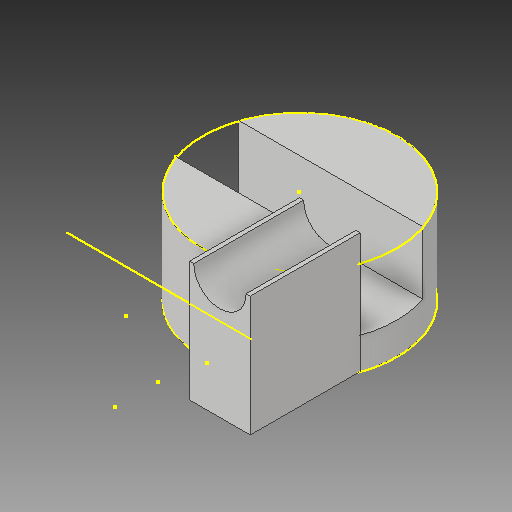
# Autodesk Inventor part: cilindro
Saved by Autodesk Inventor 2018.2 (Build 222227000, 227)
## iProperties
Created: 2016-04-06
Part Number: cilindro
Material: Genérico
Document SubType Name: Modeling
Designer: Usuario
Density: 1 g/cm^3
Appearance: Valor por defecto
Author: Usuario
Autodesk Inventor part; units mm, degrees
ref_plane "YZ Plane" through (0, 0, 0) normal (1, 0, 0) x (0, 1, 0)
ref_plane "XZ Plane" through (0, 0, 0) normal (0, 1, 0) x (-1, 0, 0)
ref_plane "XY Plane" through (0, 0, 0) normal (0, 0, 1) x (1, 0, 0)
sketch "Boceto1" plane through (0, 0, 0) normal (0, 1, 0) x (-1, 0, 0)
  circle A0 centre (0, 0) radius 46.5
  dimension "d0" = 93
  constraints: 1 centre point, 1 coincident
  measures "d0" diameter of A0
extrude "Extrusión1" add sketch "Boceto1" along normal blind 45
sketch "Boceto2" plane through (0, 0, 0) normal (0, -1, 0) x (1, 0, 0)
  point P0 (0, 0)
sketch "Boceto3" plane through (0, 45, 0) normal (0, 1, 0) x (1, 0, 0)
  line L0 (46.5, -15) -> (-46.6883, -15)
  circle A0 centre (0, 0) radius 46.5 projected
  line L1 (46.5, -15) -> (46.5, 15)
  line L2 (46.5, 0) -> (46.5, -15)
  line L3 (46.5, 0) -> (46.5, 15)
  line L4 (-46.6883, -15) -> (-46.6883, 15)
  line L5 (-46.6883, 15) -> (46.5, 15)
  constraints: 13 end point, 2 midpoint, 2 vertical, 1 horizontal, 1 horizontal alignment, 1 perpendicular, 1 point on line, 1 other
extrude "Extrusión2" cut sketch "Boceto3" against normal blind 30 contours L0 A0 L1 | L0 A0 L5 | A0 L5 L1 | L0 L4 L5 A0
sketch "Boceto4" plane through (0, 45, 0) normal (0, 1, 0) x (1, 0, 0)
  circle A0 centre (0, 0) radius 46.5 projected
  point P0 (-44.0142, -15)
  point P1 (44.0142, -15)
sketch "Boceto5" plane through (0, 45, 0) normal (0, 1, 0) x (1, 0, 0)
  line L0 (-20.0239, -77.8543) -> (-20, -77.821)
  point P0 (0, 0)
  point P1 (-20, -41.9792)
  point P2 (0, 0)
  point P3 (0, 0)
  constraints: 2 end point
extrude "Extrusión3" [suppressed]
sketch "Boceto6" plane through (0, 45, 0) normal (0, 1, 0) x (1, 0, 0)
  point P0 (0, 0)
sketch "Boceto7" plane through (0, 45, 0) normal (0, 1, 0) x (1, 0, 0)
  point P0 (0, 0)
sketch "Boceto8" plane through (0, 45, 0) normal (0, 1, 0) x (1, 0, 0)
  point P0 (0, 0)
sketch "Boceto9" plane through (0, 0, 0) normal (0, -1, 0) x (1, 0, 0)
  arc A0 (-44.0142, -15) -> (-44.0142, 15) centre (0, 0) ccw projected
  point P0 (5, 46.2304)
  point P1 (19.0142, 42.4348)
hole "Agujero1" at (0, 0, 0) direction (0, 1, 0) diameter 3.5 depth 10
sketch "Boceto10" plane through (0, 0, 0) normal (0, -1, 0) x (1, 0, 0)
  point P0 (0, 0)
sketch "Boceto11" plane through (0, 0, 0) normal (0, -1, 0) x (1, 0, 0)
  point P0 (0, 0)
sketch "Boceto12" plane through (0, 0, 0) normal (0, -1, 0) x (1, 0, 0)
  line L0 (1.5, -0.9014) -> (-1.5, -0.9014)
  arc A0 (-1.5, -0.9014) -> (1.5, -0.9014) centre (0, 0) ccw
  constraints: 2 end point, 2 point on circle, 1 centre point, 1 coincident
extrude "Extrusión4" add sketch "Boceto12" against normal blind 10
sketch "Boceto13" plane through (5, 40, 88) normal (0, 0, 1) x (1, 0, 0)
  point P0 (-5, -40)
  point P1 (39.0142, 0)
sketch "Boceto14" plane through (5, 40, 88) normal (0, 0, 1) x (1, 0, 0)
  point P0 (-5, -40)
sketch "Boceto15" plane through (5, 40, 88) normal (0, 0, 1) x (1, 0, 0)
  point P0 (-5, -40)
  point P1 (39.0142, 0)
sketch "Boceto16" plane through (5, 40, 88) normal (0, 0, 1) x (1, 0, 0)
  point P0 (-5, -40)
  point P1 (0, 0)
  point P2 (39.0142, 0)
sketch "Boceto17" plane through (5, 40, 88) normal (0, 0, 1) x (1, 0, 0)
  point P0 (-5, -40)
  point P1 (39.0586, 0)
  point P2 (0, 0)
sketch "Boceto18" plane through (5, 40, 88) normal (0, 0, 1) x (1, 0, 0)
  line L0 (0, -40) -> (0, 0) projected
  line L1 (39.0142, -40) -> (0, -40) projected
  line L2 (39.0142, 20) -> (39.0142, -40)
  line L3 (0, 20) -> (0, -40)
  line L4 (0, -40) -> (39.0142, -40)
  line L5 (0, 20) -> (2, 20)
  line L6 (39.0142, 20) -> (38, 20)
  arc A0 (2, 20) -> (38, 20) centre (20, 18.1) ccw
  point P0 (-5, -40)
  constraints: 10 end point, 2 horizontal, 2 perpendicular, 2 point on circle, 1 centre point
extrude "Extrusión5" [suppressed]
sketch "Boceto19" plane through (0, 15, 0) normal (0, 1, 0) x (1, 0, 0)
  point P0 (0, 0)
sketch "Boceto20" plane through (0, 45, 0) normal (0, 1, 0) x (1, 0, 0)
  point P0 (0, 0)
sketch "Boceto21" plane through (0, 45, 0) normal (0, 1, 0) x (1, 0, 0)
  point P0 (0, 0)
sketch "Boceto22" plane through (0, 45, 0) normal (0, 1, 0) x (1, 0, 0)
  point P0 (0, 0)
sketch "Boceto23" plane through (19.0142, 40, 67.4096) normal (0, 0, 1) x (1, 0, 0)
  line L0 (25, 0) -> (-63.0284, 0) projected
  point P0 (-19.0142, -40)
sketch "Boceto24" plane through (0, 45, 0) normal (0, 1, 0) x (1, 0, 0)
  arc A0 (-1.5, 0.9014) -> (1.5, 0.9014) centre (0, 0) ccw projected
  arc A1 (15.0142, -44.0094) -> (44.0142, -15) centre (0, 0) ccw
  circle A2 centre (0, 0) radius 46.5 projected
  arc A3 (-44.0142, -15) -> (44.0142, -15) centre (0, 0) ccw projected
  line L0 (44.0142, -15) -> (44.0142, -67.5)
  line L1 (44.0142, -67.5) -> (15.0142, -67.5)
  line L2 (15.0142, -67.5) -> (15.0142, -44.0094)
  constraints: 6 end point, 3 point on circle, 1 centre point, 1 coincident, 1 horizontal, 1 perpendicular
extrude "Extrusión6" add sketch "Boceto24" against normal blind 40 contours A1 L0 L1 L2
sketch "Boceto25" plane through (15.0142, 45, 67.5) normal (0, 0, 1) x (1, 0, 0)
  line L0 (29, 0) -> (29, 12.5)
  line L1 (29, 12.5) -> (27, 12.5)
  line L2 (0, 12.5) -> (2, 12.5)
  arc A0 (2, 12.5) -> (27, 12.5) centre (14.5, 12.5) ccw
  line L3 (29, -40) -> (0, -40) projected
  line L4 (0, 12.5) -> (0, -40)
  line L5 (0, -40) -> (29, -40)
  line L6 (29, -40) -> (29, 0)
  point P0 (0, 0)
  constraints: 12 end point, 2 perpendicular, 2 point on circle, 2 vertical, 1 centre point, 1 collinear
sketch "Boceto26" plane through (0, 45, 0) normal (0, 1, 0) x (1, 0, 0)
  point P0 (0, 0)
extrude "Extrusión7" add sketch "Boceto25" against normal blind 52.5
sketch "Boceto27" plane through (15.0142, 5, 67.5) normal (0, 0, 1) x (1, 0, 0)
  point P0 (-15.0142, -5)
sketch "Boceto28" plane through (15.0142, 5, 67.5) normal (0, 0, 1) x (1, 0, 0)
  line L0 (0, 0) -> (0, -5)
  line L1 (29, 0) -> (29, -5)
  line L2 (29, -5) -> (0, -5)
  line L3 (0, 0) -> (29, 0) projected
  line L4 (29, 0) -> (0, 0)
  point P0 (-15.0142, -5)
  constraints: 8 end point, 2 vertical, 1 horizontal, 1 perpendicular
extrude "Extrusión8" add sketch "Boceto28" against normal blind 70
